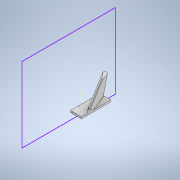
# Autodesk Inventor part: Tall KauriSpoilerFin
Saved by Autodesk Inventor 2020 (Build 240168000, 168)
## iProperties
Created: 2022-06-17
Part Number: Tall KauriSpoilerFin
Material: Generic
Document SubType Name: Modeling
Designer: Steven
Density: 1 g/cm^3
Appearance: Default
Author: Steven
Autodesk Inventor part; units mm, degrees
ref_plane "YZ Plane" through (0, 0, 0) normal (1, 0, 0) x (0, 1, 0)
ref_plane "XZ Plane" through (0, 0, 0) normal (0, 1, 0) x (-1, 0, 0)
ref_plane "XY Plane" through (0, 0, 0) normal (0, 0, 1) x (1, 0, 0)
sketch "Sketch1" plane through (0, 0, 0) normal (0, 1, 0) x (-1, 0, 0)
  circle A0 centre (0, 23) radius 1.5
  circle A1 centre (0, 0) radius 1.5
  line L0 (12, 34.0289) -> (9.7391, 34.0289)
  line L1 (9.7391, 34.0289) -> (9.7967, 35.3255)
  line L2 (9.7967, 35.3255) -> (9.8174, 35.587)
  line L3 (9.8174, 35.587) -> (9.8558, 36.8573)
  line L4 (9.8558, 36.8573) -> (2.6679, 36.8573)
  line L5 (2.6679, 36.8573) -> (2.7679, 36.8557)
  line L6 (2.7679, 36.8557) -> (2.7482, 35.6089)
  line L7 (2.6482, 35.6105) -> (2.7482, 35.6089)
  line L8 (2.6477, 35.3749) -> (2.6482, 35.6105)
  line L9 (2.6365, 34.8641) -> (2.6477, 35.3749)
  line L10 (2.7364, 34.8625) -> (2.6365, 34.8641)
  line L11 (2.7233, 34.0273) -> (2.7364, 34.8625)
  line L12 (2.6233, 34.0289) -> (2.7233, 34.0273)
  line L13 (-2.6233, 34.0289) -> (2.6233, 34.0289)
  line L14 (-2.7233, 34.0273) -> (-2.6233, 34.0289)
  line L15 (-2.7364, 34.8625) -> (-2.7233, 34.0273)
  line L16 (-2.6365, 34.8641) -> (-2.7364, 34.8625)
  line L17 (-2.6477, 35.3749) -> (-2.6365, 34.8641)
  line L18 (-2.6482, 35.6105) -> (-2.6477, 35.3749)
  line L19 (-2.6482, 35.6105) -> (-2.7482, 35.6089)
  line L20 (-2.7482, 35.6089) -> (-2.7679, 36.8557)
  line L21 (-2.6679, 36.8573) -> (-2.7679, 36.8557)
  line L22 (-2.6679, 36.8573) -> (-9.8558, 36.8573)
  line L23 (-9.8558, 36.8573) -> (-9.8174, 35.587)
  line L24 (-9.8174, 35.587) -> (-9.7967, 35.3255)
  line L25 (-9.7967, 35.3255) -> (-9.7391, 34.0289)
  line L26 (-9.7391, 34.0289) -> (-12, 34.0289)
  line L27 (-12.5, 33.5289) -> (-12.5, -9.7955)
  line L28 (-12, -10.2955) -> (-6.6596, -10.2955)
  line L29 (-6.6596, -10.2955) -> (-4.5583, -13.4923)
  line L30 (-4.5583, -13.4923) -> (-3.7396, -12.6195)
  line L31 (-3.7396, -12.6195) -> (-2.3513, -10.418)
  line L32 (-2.3513, -10.418) -> (-2.3091, -10.4026)
  line L33 (-2.3091, -10.4026) -> (-2.3069, -10.2955)
  line L34 (-2.3069, -10.2955) -> (2.3069, -10.2955)
  line L35 (2.3069, -10.2955) -> (2.3091, -10.4026)
  line L36 (2.3091, -10.4026) -> (2.3513, -10.418)
  line L37 (2.3513, -10.418) -> (3.7396, -12.6195)
  line L38 (3.7396, -12.6195) -> (4.5583, -13.4923)
  line L39 (4.5583, -13.4923) -> (6.6596, -10.2955)
  line L40 (6.6596, -10.2955) -> (12, -10.2955)
  line L41 (12.5, -9.7955) -> (12.5, 33.5289)
  line L42 (-12, 34.0289) -> (-12.5, 34.0289)
  line L43 (-12.5, 33.5289) -> (-12.5, 34.0289)
  line L44 (12, 34.0289) -> (12.5, 34.0289)
  line L45 (12.5, 33.5289) -> (12.5, 34.0289)
  line L46 (12.5, -9.7955) -> (12.5, -10.2955)
  line L47 (12, -10.2955) -> (12.5, -10.2955)
  line L48 (-12.5, -9.7955) -> (-12.5, -10.2955)
  line L49 (-12, -10.2955) -> (-12.5, -10.2955)
  constraints: 100 end point, 4 horizontal, 2 centre point, 2 vertical
extrude "Extrusion1" add sketch "Sketch1" along normal blind 3
sketch "Sketch2" plane through (12.5, 0, 33.5289) normal (1, 0, 0) x (0, 0, -1)
  line L0 (0, 0) -> (0, 3) projected
  line L1 (43.8244, 3) -> (43.8244, 3) projected
  line L2 (0, 3) -> (43.8244, 3)
  line L3 (-0.5, 3) -> (43.8244, 3) projected
  line L4 (0, 3) -> (0, 68)
  point P0 (33.5289, 0)
  dimension "d2" = 65
  constraints: 4 end point, 1 horizontal, 1 vertical
  measures "d2" distance of L0.end L4.end
sketch "Sketch3" plane through (2.3069, 0, -10.2955) normal (0, 0, -1) x (-1, 0, 0)
  line L0 (4.6137, 3) -> (8.9665, 3)
  line L1 (0, 3) -> (-4.3528, 3)
  line L2 (0, 3) -> (4.6137, 3)
  line L3 (4.9301, 3) -> (-0.3164, 3) projected
  line L4 (-4.3528, 3) -> (-29.3039, 68)
  line L5 (8.9665, 3) -> (34.9981, 68)
  line L6 (-10.1931, 3) -> (-10.1931, 68) construction
  line L7 (-10.1931, 68) -> (34.9981, 68)
  line L8 (-10.1931, 68) -> (-29.3039, 68)
  point P0 (2.3069, 0)
  dimension "d4" = 69
  constraints: 14 end point, 2 horizontal, 1 collinear
  measures "d4" angle of L2 L4
extrude "Extrusion2" [suppressed]
ref_plane "Work Plane1" through (12.5, 3, -10.2955) normal (0, 0.7071068, -0.7071068) x (-1, 0, 0)
sketch "Sketch4" plane through (12.5, 3, -10.2955) normal (0, 0.7071068, -0.7071068) x (-1, 0, 0)
  line L0 (44.6913, 77.304) -> (-19.6108, 77.304) construction
  line L1 (-19.6108, 45.9619) -> (-19.6108, 77.304) construction
  line L2 (44.6913, 45.9619) -> (-19.6108, 45.9619) construction
  line L3 (44.6913, 45.9619) -> (44.6913, 77.304) construction
  line L4 (10.1931, -2.1213) -> (14.8069, -2.1213) projected
  line L5 (14.8069, -2.1213) -> (14.8069, 0) projected
  line L6 (10.1931, 0) -> (14.8069, 0) projected
  line L7 (10.1931, -2.1213) -> (10.1931, 0) projected
  line L8 (10.1931, -2.1213) -> (10.1931, 0) projected
  line L9 (10.1931, 0) -> (14.8069, 0)
  line L10 (12.5, 0) -> (38.5316, 45.9619)
  line L11 (12.5, 0) -> (-12.4512, 45.9619)
  line L12 (19.1596, -2.1213) -> (19.1596, 0) projected
  line L13 (19.1596, 0) -> (64.3361, 79.7644)
  line L14 (5.8404, 0) -> (7.9417, -2.2605) projected
  line L15 (5.8404, 0) -> (-37.461, 79.7644)
  line L16 (-12.4512, 45.9619) -> (-30.8014, 79.7644)
  line L17 (38.5316, 45.9619) -> (57.6765, 79.7644)
  line L18 (64.3361, 79.7644) -> (57.6765, 79.7644)
  line L19 (-30.8014, 79.7644) -> (-37.461, 79.7644)
  line L20 (57.6765, 79.7644) -> (-30.8014, 79.7644) construction
  line L21 (5.8404, -2.1213) -> (5.8404, 0) projected
  line L22 (5.8404, 0) -> (19.1596, 0)
  point P0 (12.5, 5.1587)
  point P1 (12.5, 0)
  point P2 (12.5, 0)
  dimension "d13" = 50.9828
  constraints: 22 end point, 3 horizontal, 2 parallel, 2 perpendicular, 1 midpoint
  measures "d13" distance of L10.end L11.end
extrude "Extrusion5" add sketch "Sketch4" against normal up to surface contours L22 L15 L19 L16 L11 L6 | L6 L10 L17 L18 L13 L22 surface through (0, 3, 11.6825) normal (0, 1, 0)
extrude "Extrusion6" add sketch "Sketch4" along normal blind 84.5 contours L22 L15 L19 L16 L11 L6 | L6 L10 L17 L18 L13 L22
sketch "Sketch5" plane through (12.5, 0, 33.5289) normal (1, 0, 0) x (0, 0, -1)
  line L0 (28.6097, 3) -> (11.2608, 3) projected
  line L1 (43.8244, 3) -> (103.5749, 62.7505) projected
  line L2 (0, 3) -> (43.8244, 3)
  line L3 (43.8244, 3) -> (7.5719, 82.9918)
  line L4 (0, 3) -> (0, 68) projected
  line L5 (0, 68) -> (40.9338, 56.8329)
  line L6 (12.6124, 3) -> (-0.5, 3) projected
  line L7 (-3.3284, 0) -> (-3.3284, 3) projected
  line L8 (0, 3) -> (-3.3284, 3)
  line L9 (-3.3284, 3) -> (-3.3284, 0)
  line L10 (47.0212, 0) -> (47.0212, 3) projected
  line L11 (-3.3284, 0) -> (47.0212, 0)
  line L12 (47.0212, 0) -> (47.0212, 3)
  line L13 (43.8244, 3) -> (43.3244, 3) projected
  line L14 (47.0212, 3) -> (43.8244, 3)
  point P0 (33.5289, 0)
  point P1 (16.3931, 63.5278)
  constraints: 16 end point, 4 perpendicular, 2 horizontal
extrude "Extrusion7" cut sketch "Sketch5" along normal mid plane 211.75 keep common part
sketch "Sketch7" plane through (12.5, 0, -10.2955) normal (1, 0, 0) x (0, 0, -1)
  line L0 (-44.3244, 0) -> (0, 0) projected
  line L1 (0, 0) -> (0, 3) projected
  line L2 (-15.2147, 3) -> (0, 3) projected
  line L3 (-32.5636, 3) -> (-15.2147, 3) projected
  line L4 (-44.3244, 3) -> (-32.5636, 3) projected
  line L5 (-44.3244, 0) -> (-44.3244, 3) projected
  point P0 (-10.2955, 0)
extrude "Extrusion8" add sketch "Sketch7" along normal blind 4
sketch "Sketch8" plane through (-12.5, 0, 34.0289) normal (-1, 0, 0) x (0, 0, 1)
  line L0 (-44.3244, 0) -> (0, 0) projected
  line L1 (0, 0) -> (0, 3) projected
  line L2 (-13.1124, 3) -> (0, 3) projected
  line L3 (-29.7412, 3) -> (-13.1124, 3) projected
  line L4 (-44.3244, 3) -> (-29.7412, 3) projected
  line L5 (-44.3244, 0) -> (-44.3244, 3) projected
  point P0 (-34.0289, 0)
extrude "Extrusion9" add sketch "Sketch8" along normal blind 4
sketch "Sketch9" plane through (12.5, 3, -10.2955) normal (0, 0.7071068, -0.7071068) x (-1, 0, 0)
  point P0 (12.5, 5.1587)
sketch "Sketch10" plane through (16.5, 0, -10.2955) normal (1, 0, 0) x (0, 0, -1)
  line L0 (-25.635, 3) -> (-43.8244, 3) projected
  line L1 (-25.635, 3) -> (-43.8244, 18.0494)
  line L2 (-43.8244, 3) -> (-43.8244, 68) projected
  line L3 (-44.3244, 0) -> (-44.3244, 3) projected
  point P0 (-10.2955, 0)
  constraints: 2 end point, 1 point on line
extrude "Extrusion10" cut sketch "Sketch10" along normal mid plane 159.75
sketch "Sketch11" plane through (0, 3, 0) normal (0, 1, 0) x (1, 0, 0)
  line L0 (9.8404, -15.3395) -> (22.5995, -33.5289) projected
  line L1 (-23.5782, -33.5289) -> (-10.2665, -15.3395) projected
  line L2 (-10.2665, -15.3395) -> (-16.5, -15.3395) projected
  line L3 (16.5, -15.3395) -> (9.8404, -15.3395) projected
  line L4 (-16.5, 10.2955) -> (-16.5, -34.0289) projected
  line L5 (16.5, -34.0289) -> (16.5, 10.2955) projected
  point P0 (0, 0)
  point P1 (-16.5, -23.8571)
  point P2 (16.5, -24.8335)
extrude "Extrusion11" add sketch "Sketch11" against normal up to surface surface through (16.5, 3, 15.3395) normal (0, 0.7704748, -0.6374704)
sketch "Sketch12" plane through (16.5, 0, -10.2955) normal (1, 0, 0) x (0, 0, -1)
  line L0 (-45.9044, 3) -> (-47.1512, 3) projected
  line L1 (-44.3244, 0) -> (-45.621, 0) projected
  line L2 (-47.1512, 3) -> (-44.3244, 3)
  line L3 (-44.3244, 3) -> (-44.3244, 0)
  line L4 (-44.3244, 0) -> (-47.1512, 0)
  line L5 (3.1968, 0) -> (3.1968, 3) projected
  line L6 (0, 0) -> (0, 3) projected
  line L7 (3.1968, 3) -> (0, 3)
  line L8 (0, 3) -> (0, 0)
  line L9 (0, 0) -> (3.1968, 0)
  line L10 (3.1968, 0) -> (3.1968, 3)
  line L11 (-47.1528, 3) -> (-47.8658, 3)
  line L12 (-47.8658, 3) -> (-47.8658, 0)
  line L13 (-47.8658, 0) -> (-47.1528, 0)
  line L14 (-47.8658, 0) -> (-44.3244, 0)
  line L15 (-44.3244, 0) -> (-44.3244, 3) projected
  line L16 (-44.3244, 0) -> (-44.3244, 3)
  line L17 (-44.3244, 3) -> (-47.8658, 3)
  line L18 (-47.8658, 3) -> (-47.8658, 0)
  point P0 (-10.2955, 0)
  constraints: 28 end point, 7 perpendicular, 4 horizontal, 3 parallel
extrude "Extrusion12" cut sketch "Sketch12" against normal blind 159.75
fillet "Fillet1" radius 2.8 4 edges at (23.5418, 33.2639, 3.4202) (16.8822, 33.2639, 3.4202) (-17.6132, 33.2639, 3.4202) (-24.2729, 33.2639, 3.4202)
chamfer "Chamfer1" distance 4.85 distance2 15.25 1 edges at (-33.5804, 43.0247, 33.5289) measured on face at (-34.0446, 42.8388, 33.5289)
chamfer "Chamfer2" distance 4.85 distance2 15.25 1 edges at (32.1866, 43.0247, 33.5289) measured on face at (32.6534, 42.8455, 33.5289)
sketch "Sketch13" plane through (-16.5, 0, 34.0289) normal (-1, 0, 0) x (0, 0, 1)
  line L0 (-84.5082, 87.7532) -> (57.3452, 87.7532)
  line L1 (57.3452, 87.7532) -> (57.3452, -25.9852)
  line L2 (57.3452, -25.9852) -> (-84.5082, -25.9852)
  line L3 (-84.5082, -25.9852) -> (-84.5082, 87.7532)
  point P0 (-34.0289, 0)
  constraints: 8 end point, 2 parallel, 1 horizontal, 1 perpendicular
extrude "Extrusion13" cut sketch "Sketch13" against normal blind 16.5
extrude "Extrusion14" cut sketch "Sketch13" along normal blind 48.25
body "Solid1"
